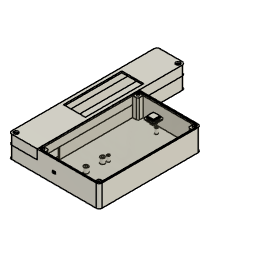
casing_doorlock (Autodesk Fusion 360 design; units mm, degrees)
Autodesk Fusion 360 part; units mm, degrees
(part 1 of 2)
sketch "Sketch1" plane through (0, 0, 0) normal (0, 0, 1) x (1, 0, 0)
  line L0 (3, 0) -> (117.6, 0)
  line L1 (120.6, 3) -> (120.6, 133.6)
  line L2 (120.6, 200) -> (3, 200)
  line L3 (0, 197) -> (0, 3)
  line L4 (0, 200) -> (-1.7, 200)
  line L5 (-1.7, 200) -> (-1.7, 201.7)
  line L6 (-1.7, 201.7) -> (0, 201.7)
  line L7 (0, 201.7) -> (0, 200)
  line L8 (120.6, 0) -> (122.3, 0)
  line L9 (122.3, 0) -> (122.3, -1.7)
  line L10 (122.3, -1.7) -> (120.6, -1.7)
  line L11 (120.6, -1.7) -> (120.6, 0)
  line L12 (118.3, -1.7) -> (2.3, -1.7)
  line L13 (-1.7, 2.3) -> (-1.7, 197.7)
  line L14 (2.3, 201.7) -> (122.3, 201.7)
  line L15 (122.3, 134.3) -> (122.3, 2.3)
  line L16 (0, 200) -> (0.3, 200)
  line L17 (0.3, 200) -> (0.3, 199.7)
  line L18 (0.3, 199.7) -> (0, 199.7)
  line L19 (0, 199.7) -> (0, 200)
  line L20 (120.6, 0) -> (120.3, 0)
  line L21 (120.3, 0) -> (120.3, 0.3)
  line L22 (120.3, 0.3) -> (120.6, 0.3)
  line L23 (120.6, 0.3) -> (120.6, 0)
  line L24 (0.3, 199.7) -> (120.3, 199.7)
  line L25 (120.3, 199.7) -> (120.3, 0.3)
  line L26 (120.3, 0.3) -> (0.3, 0.3)
  line L27 (0.3, 0.3) -> (0.3, 199.7)
  line L28 (-1.7, -1.7) -> (3.3, -1.7)
  line L29 (3.3, -1.7) -> (3.3, 3.3)
  line L30 (3.3, 3.3) -> (-1.7, 3.3)
  line L31 (-1.7, 3.3) -> (-1.7, -1.7)
  line L32 (-1.7, -1.7) -> (7.3, -1.7)
  line L33 (7.3, -1.7) -> (7.3, 5.3)
  line L34 (5.3, 7.3) -> (-1.7, 7.3)
  line L35 (-1.7, 7.3) -> (-1.7, -1.7)
  circle A0 centre (3.3, 3.3) radius 1.6
  circle A1 centre (3.3, 3.3) radius 3
  line L36 (0.3, 0.3) -> (35.3, 0.3)
  line L37 (35.3, 0.3) -> (35.3, 199.7)
  line L38 (35.3, 199.7) -> (0.3, 199.7)
  line L39 (0.3, 199.7) -> (0.3, 0.3)
  line L40 (0.3, 100) -> (35.3, 100)
  line L41 (35.3, 100) -> (35.3, 29)
  line L42 (35.3, 29) -> (0.3, 29)
  line L43 (0.3, 29) -> (0.3, 100)
  line L44 (35.3, 100) -> (0.3, 100)
  line L45 (0.3, 100) -> (0.3, 171)
  line L46 (0.3, 171) -> (35.3, 171)
  line L47 (35.3, 171) -> (35.3, 100)
  line L48 (35.3, 199.7) -> (35.6, 199.7)
  line L49 (35.6, 199.7) -> (35.6, 200)
  line L50 (35.6, 200) -> (35.3, 200)
  line L51 (35.3, 200) -> (35.3, 199.7)
  line L52 (35.6, 200) -> (35.6, 0)
  line L53 (35.6, 200) -> (37.3, 200)
  line L54 (37.3, 200) -> (37.3, 201.7)
  line L55 (37.3, 201.7) -> (35.6, 201.7)
  line L56 (35.6, 201.7) -> (35.6, 200)
  line L57 (37.3, 201.7) -> (37.3, -1.7)
  line L58 (37.3, 201.7) -> (32.3, 201.7)
  line L59 (32.3, 201.7) -> (32.3, 196.7)
  line L60 (32.3, 196.7) -> (37.3, 196.7)
  line L61 (37.3, 196.7) -> (37.3, 201.7)
  line L62 (33.3, 201.7) -> (28.3, 201.7)
  line L63 (28.3, 201.7) -> (28.3, 194.7)
  line L64 (30.3, 192.7) -> (37.3, 192.7)
  line L65 (37.3, 192.7) -> (37.3, 197.7)
  circle A2 centre (32.3, 196.7) radius 1.6
  circle A3 centre (32.3, 196.7) radius 3
  line L66 (17.8, 199.7) -> (20.8, 199.7)
  line L67 (20.8, 199.7) -> (20.8, 201.7)
  line L68 (20.8, 201.7) -> (17.8, 201.7)
  line L69 (17.8, 201.7) -> (17.8, 199.7)
  line L70 (17.8, 200) -> (14.8, 200)
  line L71 (14.8, 200) -> (14.8, 201.7)
  line L72 (14.8, 201.7) -> (17.8, 201.7)
  line L73 (17.8, 201.7) -> (17.8, 200)
  line L74 (37.3, 0) -> (40.3, 0)
  line L75 (40.3, 0) -> (40.3, 0.3)
  line L76 (40.3, 0.3) -> (37.3, 0.3)
  line L77 (37.3, 0.3) -> (37.3, 0)
  line L78 (40.3, 0) -> (40.3, 200)
  line L79 (37.3, 29) -> (40.3, 29)
  line L80 (40.3, 29) -> (40.3, 47)
  line L81 (40.3, 47) -> (37.3, 47)
  line L82 (37.3, 47) -> (37.3, 29)
  line L83 (40.3, 47) -> (120.3, 47)
  line L84 (120.3, 47) -> (120.3, 129)
  line L85 (120.3, 129) -> (40.3, 129)
  line L86 (40.3, 129) -> (40.3, 47)
  line L87 (120.3, 129) -> (120.6, 129)
  line L88 (120.6, 129) -> (120.6, 129.3)
  line L89 (120.6, 129.3) -> (120.3, 129.3)
  line L90 (120.3, 129.3) -> (120.3, 129)
  line L91 (120.6, 129.3) -> (37.3, 129.3)
  line L92 (120.6, 129.3) -> (122.3, 129.3)
  line L93 (122.3, 129.3) -> (122.3, 138.3)
  line L94 (122.3, 138.3) -> (120.6, 138.3)
  line L95 (120.6, 138.3) -> (120.6, 129.3)
  line L96 (122.3, 138.3) -> (120.6, 138.3)
  line L97 (120.6, 138.3) -> (120.6, 136.6)
  line L98 (120.6, 136.6) -> (122.3, 136.6)
  line L99 (122.3, 136.6) -> (122.3, 138.3)
  line L100 (122.3, 138.3) -> (113.3, 138.3)
  line L101 (113.3, 138.3) -> (113.3, 129.3)
  line L102 (113.3, 129.3) -> (122.3, 129.3)
  line L103 (122.3, 129.3) -> (122.3, 138.3)
  line L104 (122.3, 138.3) -> (117.3, 138.3)
  line L105 (117.3, 138.3) -> (117.3, 133.3)
  line L106 (117.3, 133.3) -> (122.3, 133.3)
  line L107 (122.3, 133.3) -> (122.3, 138.3)
  line L108 (117.6, 136.6) -> (35.6, 136.6)
  line L109 (35.6, 136.6) -> (35.6, 138.3)
  line L110 (35.6, 138.3) -> (118.3, 138.3)
  line L111 (122.3, 138.3) -> (122.3, 136.6)
  circle A4 centre (117.3, 133.3) radius 1.6
  circle A5 centre (117.3, 133.3) radius 3
  line L112 (35.6, 138.3) -> (44.6, 138.3)
  line L113 (44.6, 138.3) -> (44.6, 131.3)
  line L114 (42.6, 129.3) -> (35.6, 129.3)
  line L115 (35.6, 129.3) -> (35.6, 138.3)
  line L116 (35.6, 138.3) -> (40.6, 138.3)
  line L117 (40.6, 138.3) -> (40.6, 133.3)
  line L118 (40.6, 133.3) -> (35.6, 133.3)
  line L119 (35.6, 133.3) -> (35.6, 138.3)
  circle A6 centre (40.6, 133.3) radius 1.6
  line L120 (35.6, 0) -> (35.6, -1.7)
  line L121 (35.6, -1.7) -> (44.6, -1.7)
  line L122 (44.6, -1.7) -> (44.6, 5.3)
  line L123 (42.6, 7.3) -> (35.6, 7.3)
  line L124 (35.6, 7.3) -> (35.6, -1.7)
  line L125 (35.6, -1.7) -> (40.6, -1.7)
  line L126 (40.6, -1.7) -> (40.6, 3.3)
  line L127 (40.6, 3.3) -> (35.6, 3.3)
  line L128 (35.6, 3.3) -> (35.6, -1.7)
  circle A7 centre (40.6, 3.3) radius 1.6
  line L129 (122.3, -1.7) -> (113.3, -1.7)
  line L130 (113.3, -1.7) -> (113.3, 5.3)
  line L131 (115.3, 7.3) -> (122.3, 7.3)
  line L132 (122.3, 7.3) -> (122.3, -1.7)
  line L133 (122.3, -1.7) -> (117.3, -1.7)
  line L134 (117.3, -1.7) -> (117.3, 3.3)
  line L135 (117.3, 3.3) -> (122.3, 3.3)
  line L136 (122.3, 3.3) -> (122.3, -1.7)
  circle A8 centre (117.3, 3.3) radius 1.6
  circle A9 centre (117.3, 3.3) radius 3
  line L137 (120.3, 129) -> (70.3, 129)
  line L138 (70.3, 129) -> (70.3, 59)
  line L139 (70.3, 59) -> (120.3, 59)
  line L140 (120.3, 59) -> (120.3, 129)
  line L141 (120.6, 129.3) -> (113.3, 129.3)
  line L142 (113.3, 129.3) -> (113.3, 126.3)
  line L143 (115.3, 124.3) -> (120.6, 124.3)
  line L144 (120.6, 124.3) -> (120.6, 129.3)
  line L145 (120.3, 129) -> (118.3, 129)
  line L146 (118.3, 129) -> (118.3, 127)
  line L147 (118.3, 127) -> (120.3, 127)
  line L148 (120.3, 127) -> (120.3, 129)
  circle A10 centre (118.3, 127) radius 1
  line L149 (120.3, 59) -> (118.3, 59)
  line L150 (118.3, 59) -> (118.3, 61)
  line L151 (118.3, 61) -> (120.3, 61)
  line L152 (120.3, 61) -> (120.3, 59)
  circle A11 centre (118.3, 61) radius 1
  line L153 (120.3, 61) -> (120.6, 61)
  line L154 (120.6, 61) -> (120.6, 58)
  line L155 (120.6, 58) -> (120.3, 58)
  line L156 (120.3, 58) -> (120.3, 61)
  line L157 (120.6, 58) -> (116.3, 58)
  line L158 (114.3, 60) -> (114.3, 62)
  line L159 (116.3, 64) -> (120.6, 64)
  line L160 (120.6, 64) -> (120.6, 58)
  line L161 (70.3, 59) -> (72.3, 59)
  line L162 (72.3, 59) -> (72.3, 61)
  line L163 (72.3, 61) -> (70.3, 61)
  line L164 (70.3, 61) -> (70.3, 59)
  circle A12 centre (72.3, 61) radius 1
  line L165 (70.3, 129) -> (72.3, 129)
  line L166 (72.3, 129) -> (72.3, 127)
  line L167 (72.3, 127) -> (70.3, 127)
  line L168 (70.3, 127) -> (70.3, 129)
  circle A13 centre (72.3, 127) radius 1
  circle A14 centre (72.3, 61) radius 2
  line L169 (72.3, 129) -> (69.3, 129)
  line L170 (69.3, 129) -> (69.3, 129.3)
  line L171 (69.3, 129.3) -> (72.3, 129.3)
  line L172 (72.3, 129.3) -> (72.3, 129)
  line L173 (69.3, 129.3) -> (75.3, 129.3)
  line L174 (75.3, 129.3) -> (75.3, 125)
  line L175 (73.3, 123) -> (71.3, 123)
  line L176 (69.3, 125) -> (69.3, 129.3)
  line L177 (70.3, 129) -> (37.3, 129)
  line L178 (37.3, 129) -> (37.3, 115.5)
  line L179 (37.3, 115.5) -> (70.3, 115.5)
  line L180 (70.3, 115.5) -> (70.3, 129)
  arc A15 (-1.7, 2.3) -> (2.3, -1.7) centre (2.3, 2.3) ccw
  arc A16 (0, 3) -> (3, 0) centre (3, 3) ccw
  arc A17 (118.3, -1.7) -> (122.3, 2.3) centre (118.3, 2.3) ccw
  arc A18 (117.6, 0) -> (120.6, 3) centre (117.6, 3) ccw
  arc A19 (122.3, 134.3) -> (118.3, 138.3) centre (118.3, 134.3) ccw
  arc A20 (120.6, 133.6) -> (117.6, 136.6) centre (117.6, 133.6) ccw
  arc A21 (37.3, 197.7) -> (33.3, 201.7) centre (33.3, 197.7) ccw
  line L181 (32.3, 196.7) -> (35.6, 196.7)
  line L182 (35.6, 196.7) -> (35.6, 197)
  line L183 (32.6, 200) -> (32.3, 200)
  line L184 (32.3, 200) -> (32.3, 196.7)
  arc A22 (35.6, 197) -> (32.6, 200) centre (32.6, 197) ccw
  arc A23 (28.3, 194.7) -> (30.3, 192.7) centre (30.3, 194.7) ccw
  arc A24 (2.3, 201.7) -> (-1.7, 197.7) centre (2.3, 197.7) ccw
  arc A25 (3, 200) -> (0, 197) centre (3, 197) ccw
  arc A26 (7.3, 5.3) -> (5.3, 7.3) centre (5.3, 5.3) ccw
  arc A27 (44.6, 5.3) -> (42.6, 7.3) centre (42.6, 5.3) ccw
  arc A28 (115.3, 7.3) -> (113.3, 5.3) centre (115.3, 5.3) ccw
  arc A29 (42.6, 129.3) -> (44.6, 131.3) centre (42.6, 131.3) ccw
  arc A30 (113.3, 126.3) -> (115.3, 124.3) centre (115.3, 126.3) ccw
  line L185 (113.3, 129.3) -> (115.3, 129.3)
  line L186 (115.3, 129.3) -> (115.3, 131.3)
  line L187 (115.3, 131.3) -> (113.3, 131.3)
  line L188 (113.3, 131.3) -> (113.3, 129.3)
  circle A31 centre (115.3, 131.3) radius 2
  arc A32 (69.3, 125) -> (71.3, 123) centre (71.3, 125) ccw
  arc A33 (73.3, 123) -> (75.3, 125) centre (73.3, 125) ccw
  arc A34 (116.3, 64) -> (114.3, 62) centre (116.3, 62) ccw
  arc A35 (114.3, 60) -> (116.3, 58) centre (116.3, 60) ccw
  line L189 (-1.7, -1.7) -> (122.3, -1.7)
  line L190 (122.3, -1.7) -> (122.3, 0)
  line L191 (122.3, 0) -> (-1.7, 0)
  line L192 (-1.7, 0) -> (-1.7, -1.7)
  line L193 (60.3, 0) -> (62.3, 0)
  line L194 (62.3, 0) -> (62.3, -1.7)
  line L195 (62.3, -1.7) -> (60.3, -1.7)
  line L196 (60.3, -1.7) -> (60.3, 0)
  line L197 (62.3, -1.7) -> (58.3, -1.7)
  line L198 (58.3, -1.7) -> (58.3, 0)
  line L199 (58.3, 0) -> (62.3, 0)
  line L200 (62.3, 0) -> (62.3, -1.7)
  line L201 (37.3, 136.6) -> (37.6, 136.6)
  line L202 (37.6, 136.6) -> (37.6, 136.3)
  line L203 (37.6, 136.3) -> (37.3, 136.3)
  line L204 (37.3, 136.3) -> (37.3, 136.6)
  line L205 (37.6, 136.3) -> (120.3, 136.3)
  line L206 (120.3, 136.3) -> (120.3, 0.3)
  line L207 (120.3, 0.3) -> (37.6, 0.3)
  line L208 (37.6, 0.3) -> (37.6, 136.3)
  line L209 (40.3, 136.6) -> (44.6, 136.6)
  line L210 (44.6, 136.6) -> (44.6, 129.3)
  line L211 (44.6, 129.3) -> (37.3, 129.3)
  line L212 (37.3, 129.3) -> (37.3, 133.6)
  line L213 (40.6, 136.3) -> (44.6, 136.3)
  line L214 (44.6, 136.3) -> (44.6, 129.3)
  line L215 (44.6, 129.3) -> (37.6, 129.3)
  line L216 (37.6, 129.3) -> (37.6, 133.3)
  arc A36 (40.3, 136.6) -> (37.3, 133.6) centre (40.3, 133.6) ccw
  arc A37 (40.6, 136.3) -> (37.6, 133.3) centre (40.6, 133.3) ccw
  circle A38 centre (40.6, 3.3) radius 3
  line L217 (40.3, 0) -> (40.6, 0)
  line L218 (40.6, 0) -> (40.6, 3.3)
  line L219 (40.6, 3.3) -> (37.3, 3.3)
  line L220 (37.3, 3.3) -> (37.3, 3)
  arc A39 (37.3, 3) -> (40.3, 0) centre (40.3, 3) ccw
  line L221 (35.3, 29) -> (40.3, 29)
  line L222 (120.3, 58) -> (67.3, 58)
  line L223 (67.3, 58) -> (67.3, 29.5)
  line L224 (67.3, 29.5) -> (120.3, 29.5)
  line L225 (120.3, 29.5) -> (120.3, 58)
  line L226 (120.3, 29.5) -> (117.3, 29.5)
  line L227 (117.3, 29.5) -> (117.3, 32.5)
  line L228 (117.3, 32.5) -> (120.3, 32.5)
  line L229 (120.3, 32.5) -> (120.3, 29.5)
  circle A40 centre (117.3, 32.5) radius 1.6
  line L230 (120.6, 29.5) -> (116.3, 29.5)
  line L231 (114.3, 31.5) -> (114.3, 33.5)
  line L232 (116.3, 35.5) -> (120.6, 35.5)
  line L233 (120.6, 35.5) -> (120.6, 29.5)
  line L234 (67.3, 29.5) -> (70.3, 29.5)
  line L235 (70.3, 29.5) -> (70.3, 32.5)
  line L236 (70.3, 32.5) -> (67.3, 32.5)
  line L237 (67.3, 32.5) -> (67.3, 29.5)
  circle A41 centre (70.3, 32.5) radius 1.6
  circle A42 centre (70.3, 32.5) radius 3
  line L238 (67.3, 58) -> (70.3, 58)
  line L239 (70.3, 58) -> (70.3, 55)
  line L240 (70.3, 55) -> (67.3, 55)
  line L241 (67.3, 55) -> (67.3, 58)
  circle A43 centre (70.3, 55) radius 1.6
  circle A44 centre (70.3, 55) radius 3
  line L242 (120.3, 58) -> (117.3, 58)
  line L243 (117.3, 58) -> (117.3, 55)
  line L244 (117.3, 55) -> (120.3, 55)
  line L245 (120.3, 55) -> (120.3, 58)
  circle A45 centre (117.3, 55) radius 1.6
  line L246 (120.6, 58) -> (114.3, 58)
  line L247 (114.3, 58) -> (114.3, 54)
  line L248 (116.3, 52) -> (120.6, 52)
  line L249 (120.6, 52) -> (120.6, 58)
  line L250 (114.3, 58) -> (114.3, 62)
  arc A46 (114.3, 54) -> (116.3, 52) centre (116.3, 54) ccw
  arc A47 (116.3, 35.5) -> (114.3, 33.5) centre (116.3, 33.5) ccw
  arc A48 (114.3, 31.5) -> (116.3, 29.5) centre (116.3, 31.5) ccw
  line L251 (70.3, 129) -> (78.8, 129)
  line L252 (78.8, 129) -> (78.8, 116.5)
  line L253 (78.8, 116.5) -> (70.3, 116.5)
  line L254 (70.3, 116.5) -> (70.3, 129)
  circle A49 centre (78.8, 116.5) radius 1.8
  line L255 (78.8, 116.5) -> (75.8, 116.5)
  line L256 (75.8, 116.5) -> (75.8, 119.5)
  line L257 (75.8, 119.5) -> (78.8, 119.5)
  line L258 (78.8, 119.5) -> (78.8, 116.5)
  line L259 (76.8, 119.5) -> (80.8, 119.5)
  line L260 (81.8, 118.5) -> (81.8, 114.5)
  line L261 (80.8, 113.5) -> (76.8, 113.5)
  line L262 (75.8, 114.5) -> (75.8, 118.5)
  line L263 (78.8, 116.5) -> (74.4, 116.5)
  line L264 (74.4, 116.5) -> (74.4, 120.9)
  line L265 (74.4, 120.9) -> (78.8, 120.9)
  line L266 (78.8, 120.9) -> (78.8, 116.5)
  line L267 (75.4, 120.9) -> (82.2, 120.9)
  line L268 (83.2, 119.9) -> (83.2, 113.1)
  line L269 (82.2, 112.1) -> (75.4, 112.1)
  line L270 (74.4, 113.1) -> (74.4, 119.9)
  line L271 (74.4, 120.9) -> (73.7, 120.9)
  line L272 (73.7, 120.9) -> (73.7, 121.6)
  line L273 (73.7, 121.6) -> (74.4, 121.6)
  line L274 (74.4, 121.6) -> (74.4, 120.9)
  line L275 (74.7, 121.6) -> (82.9, 121.6)
  line L276 (83.9, 120.6) -> (83.9, 112.4)
  line L277 (82.9, 111.4) -> (74.7, 111.4)
  line L278 (73.7, 112.4) -> (73.7, 120.6)
  line L279 (78.8, 116.5) -> (71.8, 116.5)
  line L280 (71.8, 116.5) -> (71.8, 123.5)
  line L281 (71.8, 123.5) -> (78.8, 123.5)
  line L282 (78.8, 123.5) -> (78.8, 116.5)
  line L283 (73.8, 123.5) -> (83.8, 123.5)
  line L284 (85.8, 121.5) -> (85.8, 111.5)
  line L285 (83.8, 109.5) -> (73.8, 109.5)
  line L286 (71.8, 111.5) -> (71.8, 121.5)
  arc A50 (81.8, 118.5) -> (80.8, 119.5) centre (80.8, 118.5) ccw
  arc A51 (80.8, 113.5) -> (81.8, 114.5) centre (80.8, 114.5) ccw
  arc A52 (75.8, 114.5) -> (76.8, 113.5) centre (76.8, 114.5) ccw
  arc A53 (76.8, 119.5) -> (75.8, 118.5) centre (76.8, 118.5) ccw
  arc A54 (83.2, 119.9) -> (82.2, 120.9) centre (82.2, 119.9) ccw
  arc A55 (82.2, 112.1) -> (83.2, 113.1) centre (82.2, 113.1) ccw
  arc A56 (82.9, 111.4) -> (83.9, 112.4) centre (82.9, 112.4) ccw
  arc A57 (83.9, 120.6) -> (82.9, 121.6) centre (82.9, 120.6) ccw
  arc A58 (74.4, 113.1) -> (75.4, 112.1) centre (75.4, 113.1) ccw
  arc A59 (73.7, 112.4) -> (74.7, 111.4) centre (74.7, 112.4) ccw
  arc A60 (75.4, 120.9) -> (74.4, 119.9) centre (75.4, 119.9) ccw
  arc A61 (74.7, 121.6) -> (73.7, 120.6) centre (74.7, 120.6) ccw
  arc A62 (73.8, 123.5) -> (71.8, 121.5) centre (73.8, 121.5) ccw
  arc A63 (85.8, 121.5) -> (83.8, 123.5) centre (83.8, 121.5) ccw
  arc A64 (83.8, 109.5) -> (85.8, 111.5) centre (83.8, 111.5) ccw
  arc A65 (71.8, 111.5) -> (73.8, 109.5) centre (73.8, 111.5) ccw
  circle A66 centre (72.3, 127) radius 2
  line L287 (0.3, 29) -> (35.3, 29)
  line L288 (35.3, 29) -> (35.3, 69)
  line L289 (35.3, 69) -> (0.3, 69)
  line L290 (0.3, 69) -> (0.3, 29)
  line L291 (17.8, 69) -> (2.8, 69)
  line L292 (2.8, 69) -> (32.8, 69)
  line L293 (32.8, 69) -> (32.8, 149)
  line L294 (32.8, 149) -> (2.8, 149)
  line L295 (2.8, 149) -> (2.8, 69)
  point P0 (114.3, 58)
  point P1 (69.3, 123)
  point P2 (114.3, 29.5)
  point P3 (81.8, 119.5)
  point P4 (75.8, 113.5)
  point P5 (83.2, 120.9)
  point P6 (74.4, 112.1)
  point P7 (83.9, 121.6)
  point P8 (73.7, 111.4)
  point P9 (85.8, 123.5)
  point P10 (71.8, 109.5)
  dimension "d1" = 120.6
  dimension "d2" = 200
  dimension "d3" = 1.7
  dimension "d4" = 1.7
  dimension "d5" = 1.7
  dimension "d6" = 1.7
  dimension "d7" = 0.3
  dimension "d8" = 0.3
  dimension "d9" = 0.3
  dimension "d10" = 0.3
  dimension "d11" = 5
  dimension "d12" = 5
  dimension "d13" = 9
  dimension "d14" = 9
  dimension "d15" = 3.2
  dimension "d16" = 35
  dimension "d17" = 71
  dimension "d18" = 71
  dimension "d19" = 0.3
  dimension "d20" = 1.7
  dimension "d21" = 5
  dimension "d22" = 5
  dimension "d23" = 9
  dimension "d24" = 9
  dimension "d25" = 3.2
  dimension "d26" = 3
  dimension "d27" = 3
  dimension "d28" = 3
  dimension "d29" = 18
  dimension "d30" = 80
  dimension "d31" = 82
  dimension "d32" = 0.3
  dimension "d33" = 9
  dimension "d34" = 1.7
  dimension "d35" = 9
  dimension "d36" = 5
  dimension "d37" = 5
  dimension "d38" = 1.7
  dimension "d39" = 3.2
  dimension "d40" = 9
  dimension "d41" = 5
  dimension "d42" = 5
  dimension "d43" = 3.2
  dimension "d44" = 9
  dimension "d45" = 9
  dimension "d46" = 5
  dimension "d47" = 5
  dimension "d48" = 3.2
  dimension "d49" = 9
  dimension "d50" = 9
  dimension "d51" = 5
  dimension "d52" = 5
  dimension "d53" = 3.2
  dimension "d54" = 50
  dimension "d55" = 70
  dimension "d56" = 5
  dimension "d57" = 2
  dimension "d58" = 2
  dimension "d59" = 2
  dimension "d60" = 2
  dimension "d61" = 2
  dimension "d62" = 2
  dimension "d63" = 3
  dimension "d64" = 6.3
  dimension "d65" = 6
  dimension "d66" = 2
  dimension "d67" = 2
  dimension "d68" = 2
  dimension "d69" = 2
  dimension "d70" = 2
  dimension "d71" = 2
  dimension "d72" = 4
  dimension "d73" = 3
  dimension "d74" = 6
  dimension "d75" = 6.3
  dimension "d86" = 13.5
  dimension "d87" = 4
  dimension "d88" = 3
  dimension "d89" = 4
  dimension "d90" = 3
  dimension "d91" = 4
  dimension "d92" = 3
  dimension "d93" = 4
  dimension "d94" = 3
  dimension "d95" = 2
  dimension "d96" = 4
  dimension "d97" = 3
  dimension "d98" = 2
  dimension "d99" = 2
  dimension "d100" = 2
  dimension "d101" = 2
  dimension "d102" = 2
  dimension "d103" = 2
  dimension "d104" = 2
  dimension "d105" = 2
  dimension "d106" = 2
  dimension "d107" = 2
  dimension "d108" = 2
  dimension "d113" = 2
  dimension "d114" = 4
  dimension "d119" = 0.3
  dimension "d120" = 0.3
  dimension "d121" = 3
  dimension "d122" = 3
  dimension "d123" = 3
  dimension "d142" = 53
  dimension "d143" = 28.5
  dimension "d144" = 3
  dimension "d145" = 3
  dimension "d146" = 3.2
  dimension "d147" = 6.3
  dimension "d148" = 6
  dimension "d149" = 3
  dimension "d150" = 3
  dimension "d151" = 3.2
  dimension "d152" = 3
  dimension "d153" = 3
  dimension "d154" = 3.2
  dimension "d155" = 3
  dimension "d156" = 3
  dimension "d157" = 3.2
  dimension "d158" = 6.3
  dimension "d159" = 6
  dimension "d160" = 2
  dimension "d161" = 2
  dimension "d162" = 2
  dimension "d205" = 8.5
  dimension "d206" = 12.5
  dimension "d207" = 3.6
  dimension "d208" = 3
  dimension "d209" = 3
  dimension "d210" = 6
  dimension "d211" = 6
  dimension "d212" = 4.4
  dimension "d213" = 4.4
  dimension "d214" = 8.8
  dimension "d215" = 8.8
  dimension "d216" = 0.7
  dimension "d217" = 0.7
  dimension "d218" = 10.2
  dimension "d219" = 10.2
  dimension "d220" = 7
  dimension "d221" = 7
  dimension "d222" = 14
  dimension "d223" = 14
  dimension "d224" = 1
  dimension "d225" = 1
  dimension "d226" = 1
  dimension "d227" = 1
  dimension "d228" = 1
  dimension "d229" = 1
  dimension "d230" = 1
  dimension "d231" = 1
  dimension "d232" = 1
  dimension "d233" = 1
  dimension "d234" = 1
  dimension "d235" = 1
  dimension "d236" = 2
  dimension "d237" = 2
  dimension "d238" = 2
  dimension "d239" = 2
  dimension "d265" = 40
  dimension "d266" = 15
  dimension "d267" = 30
  dimension "d268" = 80
  constraint horizontal L0
  constraint vertical L1
  constraint horizontal L2
  constraint vertical L3
  constraint horizontal L4
  constraint vertical L5
  constraint horizontal L6
  constraint vertical L7
  constraint horizontal L8
  constraint vertical L9
  constraint horizontal L10
  constraint vertical L11
  constraint horizontal L12
  constraint vertical L13
  constraint horizontal L14
  constraint vertical L15
  constraint horizontal L16
  constraint vertical L17
  constraint horizontal L18
  constraint vertical L19
  constraint horizontal L20
  constraint vertical L21
  constraint horizontal L22
  constraint vertical L23
  constraint horizontal L24
  constraint vertical L25
  constraint horizontal L26
  constraint vertical L27
  constraint horizontal L28
  constraint vertical L29
  constraint horizontal L30
  constraint vertical L31
  constraint horizontal L32
  constraint vertical L33
  constraint horizontal L34
  constraint vertical L35
  constraint coincident L29.end L30.start
  constraint concentric A0 A1
  constraint tangent L26 A1
  constraint horizontal L36
  constraint vertical L37
  constraint horizontal L38
  constraint vertical L39
  constraint horizontal L40
  constraint vertical L41
  constraint horizontal L42
  constraint vertical L43
  constraint midpoint L39 L40.start
  constraint horizontal L44
  constraint vertical L45
  constraint horizontal L46
  constraint vertical L47
  constraint horizontal L48
  constraint vertical L49
  constraint horizontal L50
  constraint vertical L51
  constraint coincident L0 L52.end
  constraint perpendicular L0 L52
  constraint horizontal L53
  constraint vertical L54
  constraint horizontal L55
  constraint vertical L56
  constraint coincident L12 L57.end
  constraint perpendicular L12 L57
  constraint horizontal L58
  constraint vertical L59
  constraint horizontal L60
  constraint vertical L61
  constraint horizontal L62
  constraint vertical L63
  constraint horizontal L64
  constraint vertical L65
  constraint coincident L59.end L60.start
  constraint concentric A2 A3
  constraint tangent L37 A3
  constraint horizontal L66
  constraint vertical L67
  constraint horizontal L68
  constraint vertical L69
  constraint coincident L14 L67.end
  constraint midpoint L38 L66.start
  constraint horizontal L70
  constraint vertical L71
  constraint horizontal L72
  constraint vertical L73
  constraint coincident L14 L71.end
  constraint coincident L69 L70.start
  constraint coincident L2 L70.start
  constraint horizontal L74
  constraint vertical L75
  constraint horizontal L76
  constraint vertical L77
  constraint coincident L57 L74.start
  constraint coincident L0 L74.start
  constraint coincident L2 L78.end
  constraint perpendicular L2 L78
  constraint horizontal L79
  constraint vertical L80
  constraint horizontal L81
  constraint vertical L82
  constraint coincident L78 L80.end
  constraint coincident L57 L79.start
  constraint horizontal L83
  constraint vertical L84
  constraint horizontal L85
  constraint vertical L86
  constraint horizontal L87
  constraint vertical L88
  constraint horizontal L89
  constraint vertical L90
  constraint coincident L57 L91.end
  constraint perpendicular L57 L91
  constraint horizontal L92
  constraint vertical L93
  constraint horizontal L94
  constraint vertical L95
  constraint horizontal L96
  constraint vertical L97
  constraint horizontal L98
  constraint vertical L99
  constraint horizontal L100
  constraint vertical L101
  constraint horizontal L102
  constraint vertical L103
  constraint horizontal L104
  constraint vertical L105
  constraint horizontal L106
  constraint vertical L107
  constraint horizontal L108
  constraint vertical L109
  constraint horizontal L110
  constraint vertical L111
  constraint coincident L105.end L106.start
  constraint concentric A4 A5
  constraint tangent L25 A5
  constraint horizontal L112
  constraint vertical L113
  constraint horizontal L114
  constraint vertical L115
  constraint horizontal L116
  constraint vertical L117
  constraint horizontal L118
  constraint vertical L119
  constraint coincident L117.end L118.start
  constraint coincident L12 L120.end
  constraint perpendicular L12 L120
  constraint horizontal L121
  constraint vertical L122
  constraint horizontal L123
  constraint vertical L124
  constraint horizontal L125
  constraint vertical L126
  constraint horizontal L127
  constraint vertical L128
  constraint coincident L126.end L127.start
  constraint horizontal L129
  constraint vertical L130
  constraint horizontal L131
  constraint vertical L132
  constraint horizontal L133
  constraint vertical L134
  constraint horizontal L135
  constraint vertical L136
  constraint coincident L134.end L135.start
  constraint concentric A8 A9
  constraint tangent L25 A9
  constraint horizontal L137
  constraint vertical L138
  constraint horizontal L139
  constraint vertical L140
  constraint horizontal L141
  constraint vertical L142
  constraint horizontal L143
  constraint vertical L144
  constraint horizontal L145
  constraint vertical L146
  constraint horizontal L147
  constraint vertical L148
  constraint coincident L146.end L147.start
  constraint horizontal L149
  constraint vertical L150
  constraint horizontal L151
  constraint vertical L152
  constraint coincident L150.end L151.start
  constraint horizontal L153
  constraint vertical L154
  constraint horizontal L155
  constraint vertical L156
  constraint horizontal L157
  constraint vertical L158
  constraint horizontal L159
  constraint vertical L160
  constraint horizontal L161
  constraint vertical L162
  constraint horizontal L163
  constraint vertical L164
  constraint coincident L162.end L163.start
  constraint horizontal L165
  constraint vertical L166
  constraint horizontal L167
  constraint vertical L168
  constraint coincident L166.end L167.start
  constraint concentric A12 A14
  constraint horizontal L169
  constraint vertical L170
  constraint horizontal L171
  constraint vertical L172
  constraint horizontal L173
  constraint vertical L174
  constraint horizontal L175
  constraint vertical L176
  constraint horizontal L177
  constraint vertical L178
  constraint horizontal L179
  constraint vertical L180
  constraint coincident L28.start L13
  constraint coincident L28.start L12
  constraint tangent L13 A15
  constraint tangent L12 A15
  constraint coincident origin L0
  constraint coincident origin L3
  constraint tangent L0 A16
  constraint tangent L3 A16
  constraint coincident L9.end L15
  constraint coincident L9.end L12
  constraint tangent L15 A17
  constraint tangent L12 A17
  constraint coincident L8.start L1
  constraint coincident L8.start L0
  constraint tangent L1 A18
  constraint tangent L0 A18
  constraint coincident L93.end L110
  constraint coincident L14.end L15
  constraint tangent L110 A19
  constraint tangent L15 A19
  constraint coincident L98.end L108
  constraint coincident L2.start L1
  constraint tangent L108 A20
  constraint tangent L1 A20
  constraint coincident L54.end L62
  constraint coincident L54.end L65
  constraint tangent L62 A21
  constraint tangent L65 A21
  constraint horizontal L181
  constraint vertical L182
  constraint horizontal L183
  constraint vertical L184
  constraint coincident L49.end L182
  constraint coincident L49.end L183
  constraint tangent L182 A22
  constraint tangent L183 A22
  constraint tangent L63 A23
  constraint tangent L64 A23
  constraint coincident L5.end L14
  constraint coincident L5.end L13
  constraint tangent L14 A24
  constraint tangent L13 A24
  constraint coincident L4.start L2
  constraint coincident L4.start L3
  constraint tangent L2 A25
  constraint tangent L3 A25
  constraint tangent L33 A26
  constraint tangent L34 A26
  constraint tangent L122 A27
  constraint tangent L123 A27
  constraint tangent L130 A28
  constraint tangent L131 A28
  constraint tangent L113 A29
  constraint tangent L114 A29
  constraint tangent L142 A30
  constraint tangent L143 A30
  constraint horizontal L185
  constraint vertical L186
  constraint horizontal L187
  constraint vertical L188
  constraint coincident L186.end L187.start
  constraint coincident L185.end A31
  constraint coincident P1 L175
  constraint coincident P1 L176
  constraint tangent L175 A32
  constraint tangent L176 A32
  constraint tangent L174 A33
  constraint tangent L175 A33
  constraint tangent L158 A34
  constraint tangent L159 A34
  constraint coincident P0 L157
  constraint coincident P0 L158
  constraint tangent L157 A35
  constraint tangent L158 A35
  constraint horizontal L189
  constraint vertical L190
  constraint horizontal L191
  constraint vertical L192
  constraint horizontal L193
  constraint vertical L194
  constraint horizontal L195
  constraint vertical L196
  constraint midpoint L191 L193.start
  constraint horizontal L197
  constraint vertical L198
  constraint horizontal L199
  constraint vertical L200
  constraint horizontal L201
  constraint vertical L202
  constraint horizontal L203
  constraint vertical L204
  constraint coincident L108 L201.start
  constraint coincident L57 L201.start
  constraint horizontal L205
  constraint vertical L206
  constraint horizontal L207
  constraint vertical L208
  constraint horizontal L209
  constraint vertical L210
  constraint horizontal L211
  constraint vertical L212
  constraint coincident L91 L210.end
  constraint horizontal L213
  constraint vertical L214
  constraint horizontal L215
  constraint vertical L216
  constraint coincident L201.start L209
  constraint coincident L201.start L212
  constraint tangent L209 A36
  constraint tangent L212 A36
  constraint coincident L202.end L213
  constraint coincident L202.end L216
  constraint tangent L213 A37
  constraint tangent L216 A37
  constraint concentric A7 A38
  constraint tangent L207 A38
  constraint horizontal L217
  constraint vertical L218
  constraint horizontal L219
  constraint vertical L220
  constraint coincident L74.start L217
  constraint coincident L74.start L220
  constraint tangent L217 A39
  constraint tangent L220 A39
  constraint perpendicular L78 L221
  constraint horizontal L222
  constraint vertical L223
  constraint horizontal L224
  constraint vertical L225
  constraint horizontal L226
  constraint vertical L227
  constraint horizontal L228
  constraint vertical L229
  constraint coincident L227.end L228.start
  constraint horizontal L230
  constraint vertical L231
  constraint horizontal L232
  constraint vertical L233
  constraint coincident L1 L230.start
  constraint horizontal L234
  constraint vertical L235
  constraint horizontal L236
  constraint vertical L237
  constraint coincident L235.end L236.start
  constraint concentric A41 A42
  constraint coincident L234.end A42
  constraint horizontal L238
  constraint vertical L239
  constraint horizontal L240
  constraint vertical L241
  constraint coincident L239.end L240.start
  constraint concentric A43 A44
  constraint coincident L238.end A44
  constraint horizontal L242
  constraint vertical L243
  constraint horizontal L244
  constraint vertical L245
  constraint coincident L243.end L244.start
  constraint horizontal L246
  constraint vertical L247
  constraint horizontal L248
  constraint vertical L249
  constraint coincident P0 L246.end
  constraint tangent L247 A46
  constraint tangent L248 A46
  constraint tangent L231 A47
  constraint tangent L232 A47
  constraint coincident P2 L230
  constraint coincident P2 L231
  constraint tangent L230 A48
  constraint tangent L231 A48
  constraint horizontal L251
  constraint vertical L252
  constraint horizontal L253
  constraint vertical L254
  constraint coincident L252.end L253.start
  constraint horizontal L255
  constraint vertical L256
  constraint horizontal L257
  constraint vertical L258
  constraint horizontal L259
  constraint vertical L260
  constraint horizontal L261
  constraint vertical L262
  constraint horizontal L263
  constraint vertical L264
  constraint horizontal L265
  constraint vertical L266
  constraint horizontal L267
  constraint vertical L268
  constraint horizontal L269
  constraint vertical L270
  constraint horizontal L271
  constraint vertical L272
  constraint horizontal L273
  constraint vertical L274
  constraint horizontal L275
  constraint vertical L276
  constraint horizontal L277
  constraint vertical L278
  constraint horizontal L279
  constraint vertical L280
  constraint horizontal L281
  constraint vertical L282
  constraint horizontal L283
  constraint vertical L284
  constraint horizontal L285
  constraint vertical L286
  constraint coincident P3 L259
  constraint coincident P3 L260
  constraint tangent L259 A50
  constraint tangent L260 A50
  constraint tangent L260 A51
  constraint tangent L261 A51
  constraint coincident P4 L261
  constraint coincident P4 L262
  constraint tangent L261 A52
  constraint tangent L262 A52
  constraint coincident L256.end L259
  constraint coincident L256.end L262
  constraint tangent L259 A53
  constraint tangent L262 A53
  constraint coincident P5 L267
  constraint coincident P5 L268
  constraint tangent L267 A54
  constraint tangent L268 A54
  constraint tangent L268 A55
  constraint tangent L269 A55
  constraint tangent L276 A56
  constraint tangent L277 A56
  constraint coincident P7 L275
  constraint coincident P7 L276
  constraint tangent L275 A57
  constraint tangent L276 A57
  constraint coincident P6 L269
  constraint coincident P6 L270
  constraint tangent L269 A58
  constraint tangent L270 A58
  constraint coincident P8 L277
  constraint coincident P8 L278
  constraint tangent L277 A59
  constraint tangent L278 A59
  constraint coincident L264.end L267
  constraint coincident L264.end L270
  constraint tangent L267 A60
  constraint tangent L270 A60
  constraint coincident L272.end L275
  constraint coincident L272.end L278
  constraint tangent L275 A61
  constraint tangent L278 A61
  constraint coincident L280.end L283
  constraint coincident L280.end L286
  constraint tangent L283 A62
  constraint tangent L286 A62
  constraint coincident P9 L283
  constraint coincident P9 L284
  constraint tangent L283 A63
  constraint tangent L284 A63
  constraint tangent L284 A64
  constraint tangent L285 A64
  constraint coincident P10 L285
  constraint coincident P10 L286
  constraint tangent L285 A65
  constraint tangent L286 A65
  constraint concentric A13 A66
  constraint coincident L165.end A66
  constraint horizontal L287
  constraint vertical L288
  constraint horizontal L289
  constraint vertical L290
  constraint coincident L37 L288.end
  constraint coincident L41 L288.end
  constraint midpoint L289 L291.start
  constraint parallel L289 L291
  constraint horizontal L292
  constraint vertical L293
  constraint horizontal L294
  constraint vertical L295
  measures "d1" distance of origin L8.start
  measures "d2" distance of origin L4.start
  measures "d3" distance of L4.start L4.end
  measures "d4" distance of L4.start L6.end
  measures "d5" distance of L8.start L8.end
  measures "d6" distance of L8.start L10.end
  measures "d7" distance of L4.start L16.end
  measures "d8" distance of L4.start L18.end
  measures "d9" distance of L8.start L20.end
  measures "d10" distance of L8.start L22.end
  measures "d11" distance of L28.start L28.end
  measures "d12" distance of L28.start L30.end
  measures "d13" distance of L28.start L32.end
  measures "d14" distance of L28.start L34.end
  measures "d15" diameter of A0
  measures "d16" distance of L26.end L36.end
  measures "d17" distance of L40.start L42.end
  measures "d18" distance of L40.end L46.end
  measures "d19" distance of L37.end L48.end
  measures "d20" distance of L49.end L53.end
  measures "d21" distance of L54.end L58.end
  measures "d22" distance of L54.end L60.end
  measures "d23" distance of L54.end L62.end
  measures "d24" distance of L54.end L64.end
  measures "d25" diameter of A2
  measures "d26" distance of L66.start L66.end
  measures "d27" distance of L70.start L70.end
  measures "d28" distance of L74.start L74.end
  measures "d29" distance of L79.start L81.end
  measures "d30" distance of L80.end L83.end
  measures "d31" distance of L80.end L85.end
  measures "d32" distance of L84.end L89.end
  measures "d33" distance of L88.end L94.end
  measures "d34" distance of L93.end L98.end
  measures "d35" distance of L93.end L100.end
  measures "d36" distance of L93.end L104.end
  measures "d37" distance of L93.end L106.end
  measures "d38" distance of L98.end L93.end
  measures "d39" diameter of A4
  measures "d40" distance of L109.end L112.end
  measures "d41" distance of L109.end L116.end
  measures "d42" distance of L109.end L118.end
  measures "d43" diameter of A6
  measures "d44" distance of L120.end L121.end
  measures "d45" distance of L120.end L123.end
  measures "d46" distance of L120.end L125.end
  measures "d47" distance of L120.end L127.end
  measures "d48" diameter of A7
  measures "d49" distance of L9.end L129.end
  measures "d50" distance of L9.end L131.end
  measures "d51" distance of L9.end L133.end
  measures "d52" distance of L9.end L135.end
  measures "d53" diameter of A8
  measures "d54" distance of L84.end L137.end
  measures "d55" distance of L84.end L139.end
  measures "d56" distance of L88.end L143.end
  measures "d57" distance of L84.end L145.end
  measures "d58" distance of L84.end L147.end
  measures "d59" diameter of A10
  measures "d60" distance of L139.end L149.end
  measures "d61" distance of L139.end L151.end
  measures "d62" diameter of A11
  measures "d63" distance of L151.end L155.end
  measures "d64" distance of L154.end P0
  measures "d65" distance of L154.end L159.end
  measures "d66" distance of L138.end L161.end
  measures "d67" distance of L138.end L163.end
  measures "d68" diameter of A12
  measures "d69" distance of L137.end L165.end
  measures "d70" distance of L137.end L167.end
  measures "d71" diameter of A13
  measures "d72" diameter of A14
  measures "d73" distance of L165.end L169.end
  measures "d74" distance of L170.end L173.end
  measures "d75" distance of L170.end P1
  measures "d86" distance of L137.end L179.end
  measures "d87" radius of A15
  measures "d88" radius of A16
  measures "d89" radius of A17
  measures "d90" radius of A18
  measures "d91" radius of A19
  measures "d92" radius of A20
  measures "d93" radius of A21
  measures "d94" radius of A22
  measures "d95" radius of A23
  measures "d96" radius of A24
  measures "d97" radius of A25
  measures "d98" radius of A26
  measures "d99" radius of A27
  measures "d100" radius of A28
  measures "d101" radius of A29
  measures "d102" radius of A30
  measures "d103" distance of L101.end L185.end
  measures "d104" distance of L101.end L187.end
  measures "d105" radius of A32
  measures "d106" radius of A33
  measures "d107" radius of A34
  measures "d108" radius of A35
  measures "d113" distance of L193.start L193.end
  measures "d114" distance of L194.end L197.end
  measures "d119" distance of L201.start L201.end
  measures "d120" distance of L201.start L203.end
  measures "d121" radius of A36
  measures "d122" radius of A37
  measures "d123" radius of A39
  measures "d142" distance of L155.end L222.end
  measures "d143" distance of L155.end L224.end
  measures "d144" distance of L224.end L226.end
  measures "d145" distance of L224.end L228.end
  measures "d146" diameter of A40
  measures "d147" distance of L230.start P2
  measures "d148" distance of L230.start L232.end
  measures "d149" distance of L223.end L234.end
  measures "d150" distance of L223.end L236.end
  measures "d151" diameter of A41
  measures "d152" distance of L222.end L238.end
  measures "d153" distance of L222.end L240.end
  measures "d154" diameter of A43
  measures "d155" distance of L155.end L242.end
  measures "d156" distance of L155.end L244.end
  measures "d157" diameter of A45
  measures "d158" distance of L154.end P0
  measures "d159" distance of L154.end L248.end
  measures "d160" radius of A46
  measures "d161" radius of A47
  measures "d162" radius of A48
  measures "d205" distance of L137.end L251.end
  measures "d206" distance of L137.end L253.end
  measures "d207" diameter of A49
  measures "d208" distance of L252.end L255.end
  measures "d209" distance of L252.end L257.end
  measures "d210" distance of L256.end P3
  measures "d211" distance of L256.end P4
  measures "d212" distance of L252.end L263.end
  measures "d213" distance of L252.end L265.end
  measures "d214" distance of L264.end P5
  measures "d215" distance of L264.end P6
  measures "d216" distance of L264.end L271.end
  measures "d217" distance of L264.end L273.end
  measures "d218" distance of L272.end P7
  measures "d219" distance of L272.end P8
  measures "d220" distance of L252.end L279.end
  measures "d221" distance of L252.end L281.end
  measures "d222" distance of L280.end P9
  measures "d223" distance of L280.end P10
  measures "d224" radius of A50
  measures "d225" radius of A51
  measures "d226" radius of A52
  measures "d227" radius of A53
  measures "d228" radius of A54
  measures "d229" radius of A55
  measures "d230" radius of A56
  measures "d231" radius of A57
  measures "d232" radius of A58
  measures "d233" radius of A59
  measures "d234" radius of A60
  measures "d235" radius of A61
  measures "d236" radius of A62
  measures "d237" radius of A63
  measures "d238" radius of A64
  measures "d239" radius of A65
  measures "d265" distance of L42.end L289.end
  measures "d266" distance of L291.start L291.end
  measures "d267" distance of L291.end L292.end
  measures "d268" distance of L291.end L294.end